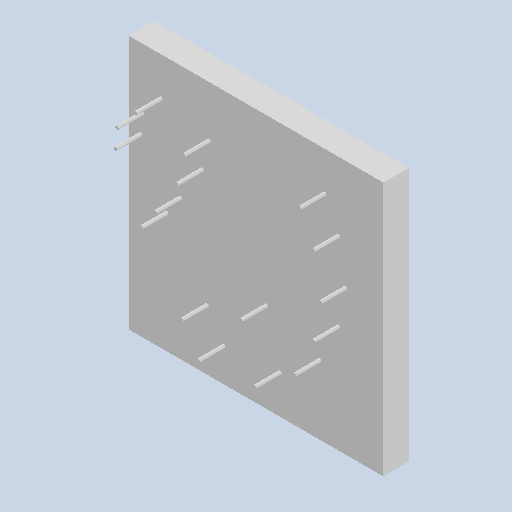
# Autodesk Inventor part: Part9
Saved by Autodesk Inventor 2025 (Build 290162010, 162A)
## iProperties
Created: 2024-07-16
Part Number: Part9
Material: Generic
Document SubType Name: Modeling
Designer: ffogue
Density: 1 g/cm^3
Appearance: Default
Author: ffogue
Autodesk Inventor part; units mm, degrees
ref_plane "YZ Plane" through (0, 0, 0) normal (1, 0, 0) x (0, 1, 0)
ref_plane "XZ Plane" through (0, 0, 0) normal (0, 1, 0) x (-1, 0, 0)
ref_plane "XY Plane" through (0, 0, 0) normal (0, 0, 1) x (1, 0, 0)
sketch "Sketch1" plane through (0, 0, 0) normal (0, 0, 1) x (1, 0, 0)
  line L0 (-1000, 1000) -> (1000, 1000)
  line L1 (1000, 1000) -> (1000, -1000)
  line L2 (1000, -1000) -> (-1000, -1000)
  line L3 (-1000, -1000) -> (-1000, 1000)
  line L4 (-1000, 1000) -> (1000, -1000) construction
  line L5 (1000, 1000) -> (-1000, -1000) construction
  point P0 (0, 0)
  dimension "d0" = 2000
  dimension "d1" = 2000
  constraints: 12 end point, 2 midpoint, 2 parallel, 1 horizontal, 1 perpendicular
  measures "d0" distance of L1.end L2.end
  measures "d1" distance of L0.end L1.end
extrude "Extrusion1" add sketch "Sketch1" along normal blind 200
sketch "Sketch2" plane through (0, 0, 200) normal (0, 0, 1) x (1, 0, 0)
  circle A0 centre (-746.6113, 699.1613) radius 13.5
  point P0 (0, 0)
  dimension "d4" = 27
  constraints: 1 centre point
  measures "d4" diameter of A0
extrude "Extrusion2" add sketch "Sketch2" along normal blind 200
pattern_sketch "Sketch Driven Pattern1" of "Extrusion2" from (-746.6113, 699.1613, 200) copies at (-368.7113, 600.7756, 200) at (540.698, 695.0149, 200) at (649.0732, 461.7726, 200) at (705.6168, 136.647, 200) at (649.0732, -155.4949, 200) at (500.6463, -459.4166, 200) at (189.6566, -697.3709, 200) at (-253.2681, -739.7786, 200) at (-385.2032, -527.7401, 200) at (81.2814, -296.8538, 200) at (-422.8989, 376.9572, 200) at (-592.5297, 101.3073, 200) at (-700.9049, -56.5436, 200) at (-893.617, 526.0067, 200) at (-905.6018, 376.9572, 200)
sketch "Sketch3" plane through (0, 0, 200) normal (0, 0, 1) x (1, 0, 0)
  point P0 (-368.7113, 600.7756)
  point P1 (175.5207, 631.4034)
  point P2 (540.698, 695.0149)
  point P3 (649.0732, 461.7726)
  point P4 (705.6168, 136.647)
  point P5 (649.0732, -155.4949)
  point P6 (500.6463, -459.4166)
  point P7 (189.6566, -697.3709)
  point P8 (-253.2681, -739.7786)
  point P9 (-385.2032, -527.7401)
  point P10 (81.2814, -296.8538)
  point P11 (-422.8989, 376.9572)
  point P12 (-592.5297, 101.3073)
  point P13 (-700.9049, -56.5436)
  point P14 (-893.617, 526.0067)
  point P15 (-905.6018, 376.9572)
body "Solid1"
